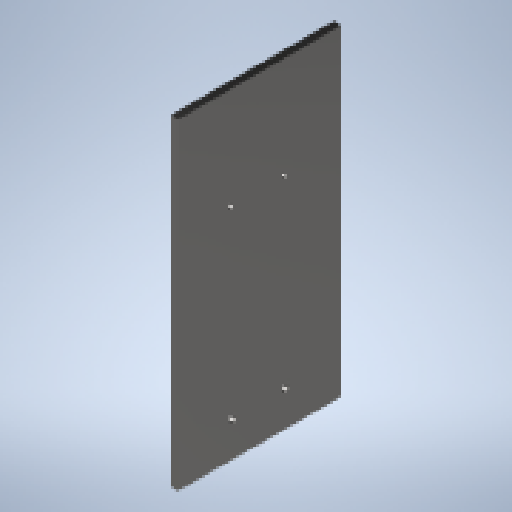
# Autodesk Inventor part: Z_Gantry_Plate
Saved by Autodesk Inventor 2023 (Build 270158000, 158)
## iProperties
Created: 2022-05-07
Part Number: Z_Gantry_Plate
Material: Steel, Mild
Document SubType Name: Modeling
Designer: plebbb
Density: 7.85 g/cm^3
Appearance: Semi-Polished
Mass: 1924.24 g
Surface Area: 706.63 cm^2
Volume: 245.125 cm^3
Author: plebbb
Autodesk Inventor part; units mm, degrees
ref_plane "YZ Plane" through (0, 0, 0) normal (1, 0, 0) x (0, 1, 0)
ref_plane "XZ Plane" through (0, 0, 0) normal (0, 1, 0) x (-1, 0, 0)
ref_plane "XY Plane" through (0, 0, 0) normal (0, 0, 1) x (1, 0, 0)
sketch "Sketch1" plane through (0, 0, 0) normal (1, 0, 0) x (0, 1, 0)
  line L0 (0, 0) -> (212.4, 0)
  line L1 (212.4, 0) -> (212.4, -142)
  line L2 (212.4, -142) -> (0, -142)
  line L3 (0, -142) -> (0, 0)
  dimension "d0" = 212.4
  dimension "d1" = 142
  constraints: 8 end point, 2 parallel, 1 horizontal, 1 perpendicular
  measures "d0" distance of L1.end L2.end
  measures "d1" distance of L0.end L1.end
extrude "Extrusion1" add sketch "Sketch1" along normal blind 6.5532
sketch "Sketch2" plane through (6.5532, 0, 0) normal (1, 0, 0) x (0, 0, -1)
  line L0 (0, 0) -> (142, 0) construction
  line L1 (48, 32) -> (94, 32) construction
  circle A0 centre (48, 32) radius 4
  circle A1 centre (94, 32) radius 4
  point P0 (71, 0)
  point P1 (71, 32)
  point P2 (71, 0)
  point P3 (71, 0)
  dimension "d9" = 8
  dimension "d10" = 46
  dimension "d11" = 32
  constraints: 4 midpoint, 2 centre point, 2 coincident, 2 end point, 1 equal radius, 1 horizontal, 1 vertical alignment
  measures "d9" diameter of A1
  measures "d10" distance of L1.start L1.end
  measures "d11" distance from line of point (71, 0) L1
extrude "Extrusion2" cut sketch "Sketch2" against normal blind 7.62
sketch "Sketch3" plane through (0, 212.4, 0) normal (0, 1, 0) x (1, 0, 0)
  line L0 (0, 142) -> (0, 0) projected
  line L1 (0, 0) -> (6.5532, 0) projected
  line L2 (6.5532, 142) -> (6.5532, 0) projected
  line L3 (0, 142) -> (6.5532, 142) projected
  point P0 (0, 0)
extrude "Extrusion3" add sketch "Sketch3" along normal blind 67.056
sketch "Sketch4" plane through (6.5532, 0, 0) normal (1, 0, 0) x (0, 0, -1)
  circle A0 centre (92.7061, 191.9341) radius 3 projected
  circle A1 centre (46.7064, 191.7587) radius 3 projected
  point P0 (0, 0)
extrude "Extrusion4" cut sketch "Sketch4" against normal blind 25.4
body "Solid1"
